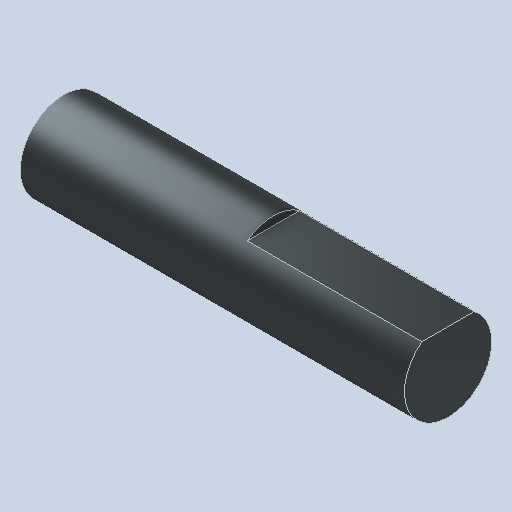
# Autodesk Inventor part: motor-shaft
Saved by Autodesk Inventor 2023 (Build 270158000, 158)
## iProperties
Created: 2022-10-02
Part Number: motor-shaft
Material: Iron, Cast
Document SubType Name: Modeling
Designer: carso
Density: 7.15 g/cm^3
Appearance: Iron Gray
Author: carso
Autodesk Inventor part; units mm, degrees
ref_plane "YZ Plane" through (0, 0, 0) normal (1, 0, 0) x (0, 1, 0)
ref_plane "XZ Plane" through (0, 0, 0) normal (0, 1, 0) x (-1, 0, 0)
ref_plane "XY Plane" through (0, 0, 0) normal (0, 0, 1) x (1, 0, 0)
sketch "Sketch1" plane through (0, 0, 0) normal (1, 0, 0) x (0, 1, 0)
  circle A0 centre (0, 0) radius 2.5
  dimension "d0" = 5
  constraints: 1 centre point, 1 coincident
  measures "d0" diameter of A0
extrude "Extrusion1" add sketch "Sketch1" along normal blind 22
sketch "Sketch2" plane through (22, 0, 0) normal (1, 0, 0) x (0, 0, -1)
  circle A0 centre (0, 0) radius 2.5 projected
  line L0 (0, -2.5) -> (0, 2)
  line L1 (0, 2) -> (-1.5, 2)
  line L2 (1.5, 2) -> (0, 2)
  dimension "d3" = 4.5
  constraints: 6 end point, 3 point on circle, 1 collinear, 1 perpendicular, 1 point on line, 1 vertical
  measures "d3" distance of L0.start L0.end
extrude "Extrusion2" cut sketch "Sketch2" against normal blind 10 contours L2 L1 A0
body "Solid1"
